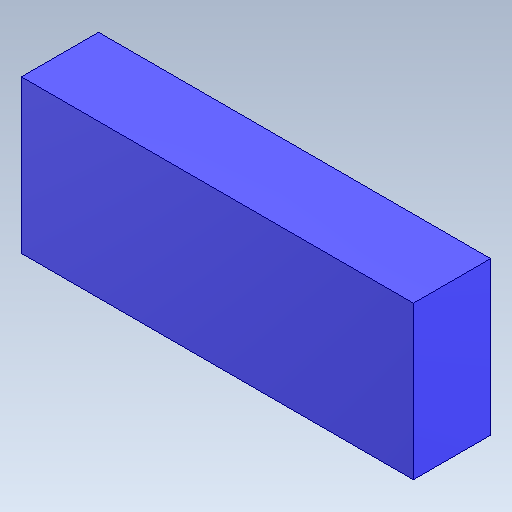
# Autodesk Inventor part: 2
Saved by Autodesk Inventor 2020 (Build 240168000, 168)
## iProperties
Created: 2019-05-24
Part Number: 2
Material: Generic
Document SubType Name: Modeling
Designer: psrob
Density: 1 g/cm^3
Appearance: 1X02_LOCK_LONGPADS, 2
Author: psrob
Autodesk Inventor part; units mm, degrees
ref_plane "YZ Plane" through (0, 0, 0) normal (1, 0, 0) x (0, 1, 0)
ref_plane "XZ Plane" through (0, 0, 0) normal (0, 1, 0) x (-1, 0, 0)
ref_plane "XY Plane" through (0, 0, 0) normal (0, 0, 1) x (1, 0, 0)
sketch "1X02_LOCK_LONGPADS, 2_34" plane through (0, 0, 0) normal (0, 0, 1) x (1, 0, 0)
  line L0 (-1.27, 0.9906) -> (3.81, 0.9906)
  line L1 (3.81, 0.9906) -> (3.81, -0.9906)
  line L2 (3.81, -0.9906) -> (-1.27, -0.9906)
  line L3 (-1.27, -0.9906) -> (-1.27, 0.9906)
  constraints: 8 end point
extrude "Extrusion1" add sketch "1X02_LOCK_LONGPADS, 2_34" along normal blind 1
body "Solid1"
